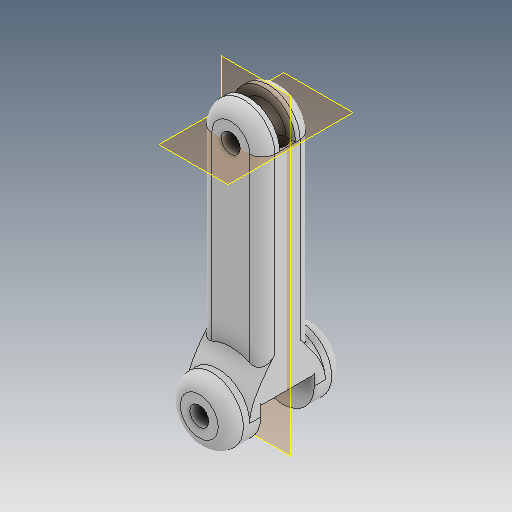
# Autodesk Inventor part: pinky_f1
Saved by Autodesk Inventor 2020.2 (Build 242310000, 310)
## iProperties
Created: 2020-04-08
Part Number: pinky_f1
Material: Generic
Document SubType Name: Modeling
Designer: Bardo91
Density: 1 g/cm^3
Appearance: Default
Author: Bardo91
Autodesk Inventor part; units mm, degrees
ref_plane "YZ Plane" through (0, 0, 0) normal (1, 0, 0) x (0, 1, 0)
ref_plane "XY Plane" through (0, 0, 0) normal (0, 0, 1) x (1, 0, 0)
sketch "Sketch1" plane through (0, 0, 0) normal (0, 0, 1) x (1, 0, 0)
  circle A0 centre (0, 0) radius 1.5
  line L0 (0, 0) -> (0, 35)
  circle A1 centre (0, 35) radius 1.5
  circle A2 centre (0, 35) radius 5
  circle A3 centre (0, 0) radius 5
  line L1 (-5, 35) -> (-5, 0)
  line L2 (5, 0) -> (5, 35)
  point P0 (0, 30)
  point P1 (0, 5)
  dimension "d0" = 3
  dimension "d1" = 35
  dimension "d2" = 3
  dimension "d3" = 10
  dimension "d4" = 10
  constraints: 6 end point, 4 centre point, 4 coincident, 4 point on circle, 2 tangent, 2 vertical
  measures "d0" diameter of A0
  measures "d1" distance of L0.start L0.end
  measures "d2" diameter of A1
  measures "d3" diameter of A2
  measures "d4" diameter of A3
extrude "base" add sketch "Sketch1" along normal blind 8
sketch "Sketch2" plane through (0, 0, 8) normal (0, 0, 1) x (1, 0, 0)
  circle A0 centre (0, 0) radius 1.5 projected
  circle A1 centre (0, 0) radius 5
  circle A2 centre (0, 0) radius 1.5
  dimension "d7" = 10
  dimension "d8" = 3
  constraints: 2 centre point, 2 coincident
  measures "d7" diameter of A1
  measures "d8" diameter of A2
extrude "joint" add sketch "Sketch2" along normal blind 5
ref_plane "Work Plane1" through (0, 0, 4) normal (0, 0, 1) x (1, 0, 0)
mirror "Mirror1" about plane through (0, 0, 4) normal (0, 0, 1) of "joint"
chamfer "Chamfer1" distance 2 angle 45 2 edges at (0, 5, 8) (0, 5, 0)
sketch "Sketch3" plane through (0, 0, 4) normal (0, 0, 1) x (1, 0, 0)
  circle A0 centre (0, 0) radius 5.25
  circle A1 centre (0, 0) radius 1.5
  dimension "d12" = 10.5
  dimension "d13" = 3
  constraints: 2 centre point, 2 coincident
  measures "d12" diameter of A0
  measures "d13" diameter of A1
extrude "joint_2" cut sketch "Sketch3" along normal mid plane 8.5
fillet "Fillet2" radius 2 8 edges at (-5, 0, 13) (-5, 0, -5) (-5, 19.9495, 0) (5, 19.9495, 0) (0, 40, 0) (0, 40, 8) (-5, 19.9495, 8) (5, 19.9495, 8)
sketch "Sketch4" plane through (0, 0, 0) normal (0, 1, 0) x (-1, 0, 0)
  line L0 (-1.5, 8.25) -> (1.5, 8.25) projected
  line L1 (0, 8.25) -> (0, -0.2496)
  line L2 (0, 4.0002) -> (-3.5, 4.0002)
  line L3 (0, 4.0002) -> (3.5, 4.0002)
  circle A0 centre (-3.5, 4.0002) radius 1.25
  circle A1 centre (3.5, 4.0002) radius 1.25
  point P0 (0, 0)
  dimension "d20" = 3.5
  dimension "d21" = 3.5
  dimension "thread_hole" = 2.5
  dimension "d23" = 2.5
  constraints: 6 end point, 2 centre point, 2 coincident, 2 horizontal, 2 midpoint, 1 vertical
  measures "d20" distance of L2.start L2.end
  measures "d21" distance of L2.start L3.end
  measures "thread_hole" diameter of A0
  measures "d23" diameter of A1
extrude "thread_hole" cut sketch "Sketch4" along normal through all
ref_plane "Work Plane2" through (5, 35, 2) normal (0, 1, 0) x (-1, 0, 0)
sketch "Sketch5" plane through (5, 35, 2) normal (0, 1, 0) x (-1, 0, 0)
  line L0 (0, -2.25) -> (10, -2.25) projected
  line L1 (5, -2.25) -> (5, 6.25)
  line L2 (10, 6.25) -> (0, 6.25) projected
  line L3 (5, 2) -> (1.5, 2)
  circle A0 centre (1.5, 2) radius 1.25
  line L4 (1.5, 0.75) -> (0, 0.75)
  line L5 (1.5, 3.25) -> (0, 3.25)
  line L6 (0, 6.25) -> (0, -2.25) projected
  line L7 (0, 3.25) -> (0, 0.75)
  point P0 (5, -2)
  dimension "d26" = 3.5
  dimension "d27" = 2.5
  constraints: 10 end point, 3 horizontal, 3 midpoint, 2 point on circle, 1 centre point, 1 coincident, 1 perpendicular, 1 point on line, 1 tangent
  measures "d26" distance of L3.start L3.end
  measures "d27" diameter of A0
revolve "thread_hole_end" cut sketch "Sketch5" angle 180 about axis through (0, 35, -0.25) along (0, 0, 1) contours L6 L5 A0 L4 | A0
sketch "Sketch6" plane through (-5, 35, 2.75) normal (0, 1, 0) x (1, 0, 0)
  arc A0 (1.5, -2.5) -> (1.5, 0) centre (1.5, -1.25) ccw projected
  line L0 (1.5, 0) -> (0, 0)
  line L1 (0, 3) -> (0, -5.5) projected
  line L2 (1.4764, -2.5) -> (0, -2.5) projected
  line L3 (0, 0) -> (0, -2.5)
  line L4 (0, -2.5) -> (1.5, -2.5)
  point P0 (1.5, -2.5)
  point P1 (1.4764, -2.5)
  constraints: 6 end point, 2 perpendicular, 1 horizontal, 1 point on line
extrude "thread_hole_end_2" cut sketch "Sketch6" against normal blind 5
equation "\"d23\" = thread_hole"
equation "\"d27\" = thread_hole"
body "Solid1"
